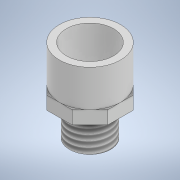
# Autodesk Inventor part: ACOPLE
Saved by Autodesk Inventor 2022 (Build 260153000, 153)
## iProperties
Created: 2022-09-01
Part Number: ACOPLE
Material: Genérico
Document SubType Name: Modeling
Designer: Usuario
Density: 1 g/cm^3
Appearance: Valor por defecto
Author: Usuario
Autodesk Inventor part; units mm, degrees
ref_plane "YZ Plane" through (0, 0, 0) normal (1, 0, 0) x (0, 1, 0)
ref_plane "XZ Plane" through (0, 0, 0) normal (0, 1, 0) x (-1, 0, 0)
ref_plane "XY Plane" through (0, 0, 0) normal (0, 0, 1) x (1, 0, 0)
sketch "Boceto1" plane through (0, 0, 0) normal (0, 1, 0) x (-1, 0, 0)
  circle A0 centre (0, 0) radius 10.7
  circle A1 centre (0, 0) radius 13.88
  dimension "d0" = 21.4
  dimension "d1" = 27.76
  constraints: 2 centre point, 2 coincident
  measures "d0" diameter of A0
  measures "d1" diameter of A1
extrude "Extrusión1" add sketch "Boceto1" against normal blind 22.6
sketch "Boceto2" plane through (0, -22.6, 0) normal (0, -1, 0) x (1, 0, 0)
  circle A0 centre (0, 0) radius 13.88 projected
  line L0 (0, -13.88) -> (-5.75, -13.88)
  line L1 (0, -13.88) -> (5.75, -13.88)
  line L2 (13.88, 0) -> (13.88, -5.75)
  line L3 (13.88, 0) -> (13.88, 5.75)
  line L4 (0, 13.88) -> (5.75, 13.88)
  line L5 (0, 13.88) -> (-5.75, 13.88)
  line L6 (-13.88, 0) -> (-13.88, -5.75)
  line L7 (-13.88, 0) -> (-13.88, 5.75)
  line L8 (-13.88, 5.75) -> (-5.75, 13.88)
  line L9 (5.75, 13.88) -> (13.88, 5.75)
  line L10 (13.88, -5.75) -> (5.75, -13.88)
  line L11 (-5.75, -13.88) -> (-13.88, -5.75)
  dimension "d5" = 5.75
  dimension "d6" = 5.75
  dimension "d7" = 5.75
  dimension "d8" = 5.75
  dimension "d9" = 5.75
  dimension "d10" = 5.75
  dimension "d11" = 5.75
  dimension "d12" = 5.75
  constraints: 24 end point, 6 tangent, 4 point on circle, 4 vertical, 3 horizontal, 1 point on line
  measures "d5" distance of L0.start L0.end
  measures "d6" distance of L0.start L1.end
  measures "d7" distance of L2.start L2.end
  measures "d8" distance of L2.start L3.end
  measures "d9" distance of L4.start L4.end
  measures "d10" distance of L4.start L5.end
  measures "d11" distance of L6.start L6.end
  measures "d12" distance of L6.start L7.end
extrude "Extrusión2" add sketch "Boceto2" against normal blind 5.97
ref_plane "Plano de trabajo2" through (0, -18.5, 0) normal (0, 1, 0) x (1, 0, 0)
sketch "Boceto4" plane through (0, -18.5, 0) normal (0, 1, 0) x (1, 0, 0)
  circle A0 centre (0, 0) radius 6.8
  dimension "d18" = 13.6
  constraints: 1 centre point, 1 coincident
  measures "d18" diameter of A0
extrude "Extrusión4" add sketch "Boceto4" against normal blind 18.97
sketch "Boceto5" plane through (0, 0, 0) normal (0, 1, 0) x (1, 0, 0)
  circle A0 centre (0, 0) radius 10.7
  constraints: 1 centre point, 1 coincident
extrude "Extrusión5" cut sketch "Boceto5" against normal blind 18.97
sketch "Boceto6" plane through (0, -37.47, 0) normal (0, -1, 0) x (1, 0, 0)
  circle A0 centre (0, 0) radius 6.7
  circle A1 centre (0, 0) radius 9.3
  dimension "d25" = 13.4
  dimension "d26" = 18.6
  constraints: 2 centre point, 2 coincident
  measures "d25" diameter of A0
  measures "d26" diameter of A1
extrude "Extrusión6" add sketch "Boceto6" against normal blind 18.97
sketch "Boceto7" plane through (0, -37.47, 0) normal (0, -1, 0) x (1, 0, 0)
  circle A0 centre (0, 0) radius 6.8
  dimension "d29" = 13.6
  constraints: 1 centre point, 1 coincident
  measures "d29" diameter of A0
extrude "Extrusión7" cut sketch "Boceto7" against normal blind 18.97
thread "Rosca2" size "M20x2.5" class "6g" standard "ANSI Metric M Profile" full length
